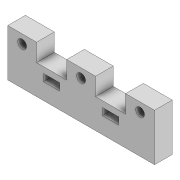
# Autodesk Inventor part: SideBoardTest
Saved by Autodesk Inventor 2022 (Build 260153000, 153)
## iProperties
Created: 2022-08-02
Part Number: SideBoardTest
Material: Generic
Document SubType Name: Modeling
Designer: wanghaoran
Density: 1 g/cm^3
Appearance: Default
Author: wanghaoran
Autodesk Inventor part; units mm, degrees
ref_plane "YZ Plane" through (0, 0, 0) normal (1, 0, 0) x (0, 1, 0)
ref_plane "XZ Plane" through (0, 0, 0) normal (0, 1, 0) x (-1, 0, 0)
ref_plane "XY Plane" through (0, 0, 0) normal (0, 0, 1) x (1, 0, 0)
sketch "Sketch1" plane through (0, 0, 0) normal (0, 0, 1) x (1, 0, 0)
  line L0 (0, 0) -> (9.8, 0)
  line L1 (9.8, 0) -> (9.8, 6)
  line L2 (9.8, 6) -> (0, 6)
  line L3 (0, 6) -> (0, 0)
  line L4 (29.8, 6) -> (20, 6)
  line L5 (20, 6) -> (20, 0)
  line L6 (20, 0) -> (29.8, 0)
  line L7 (29.8, 0) -> (29.8, 6)
  line L8 (49.8, 6) -> (40, 6)
  line L9 (40, 6) -> (40, 0)
  line L10 (40, 0) -> (49.8, 0)
  line L11 (49.8, 0) -> (49.8, 6)
  circle A0 centre (4.9, 3) radius 1.5
  circle A1 centre (24.9, 3) radius 1.5
  circle A2 centre (44.9, 3) radius 1.5
  line L12 (0, 0) -> (49.8, 0)
  line L13 (49.8, 0) -> (49.8, -10)
  line L14 (49.8, -10) -> (0, -10)
  line L15 (0, -10) -> (0, 0)
  line L16 (12.15, -2) -> (17.65, -2)
  line L17 (17.65, -2) -> (17.65, -4.4)
  line L18 (17.65, -4.4) -> (12.15, -4.4)
  line L19 (12.15, -4.4) -> (12.15, -2)
  line L20 (32.15, -2) -> (37.65, -2)
  line L21 (37.65, -2) -> (37.65, -4.4)
  line L22 (37.65, -4.4) -> (32.15, -4.4)
  line L23 (32.15, -4.4) -> (32.15, -2)
  point P0 (40, 0)
  point P1 (20, 0)
  dimension "d0" = 6
  dimension "d1" = 9.8
  dimension "d4" = 20
  dimension "d9" = 3
  dimension "d12" = 20
  dimension "d17" = 10
  dimension "d20" = 5.5
  dimension "d21" = 2.4
  dimension "d22" = 2.35
  dimension "d23" = 8
  dimension "d24" = 3
  dimension "d27" = 20
  constraints: 48 end point, 6 horizontal, 6 parallel, 3 centre point, 3 perpendicular, 2 collinear, 26 other
  measures "d0" distance of L2.end L0.start
  measures "d1" distance of L1.end L2.end
  measures "d4" distance of L1.end L4.start
  measures "d9" diameter of A0
  measures "d12" distance of A0.centre A1.centre
  measures "d17" distance of L12.end L13.end
  measures "d20" distance of L17.end L18.end
  measures "d21" distance of L16.end L17.end
  measures "d22" distance between parallel lines of L1 L19
  measures "d23" distance between parallel lines of L2 L16
  measures "d24" distance from line of L2 A0.centre
  measures "d27" distance of L16.start L20.start
extrude "Extrusion1" add sketch "Sketch1" along normal blind 6
body "Solid1"
